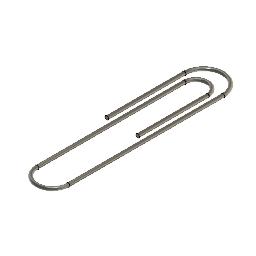
Semana2_Desafio5 v1 (Autodesk Fusion 360 design; units mm, degrees)
Autodesk Fusion 360 part; units mm, degrees
sketch "Sketch6" plane through (0, 0, 0) normal (0, 0, 1) x (1, 0, 0)
  line L0 (0, 0) -> (0, 50)
  arc A0 (25, 50) -> (0, 50) centre (12.5, 50) ccw
  line L1 (25, 50) -> (25, -50)
  arc A1 (5, -50) -> (25, -50) centre (15, -50) ccw
  line L2 (5, -50) -> (5, 45)
  arc A2 (20, 45) -> (5, 45) centre (12.5, 45) ccw
  line L3 (20, 45) -> (20, 0)
  constraint coincident L0.start origin
  constraint vertical L0
  constraint tangent L0 A0
  constraint tangent A0 L1
  constraint parallel L0 L1
  constraint tangent L1 A1
  constraint tangent A1 L2
  constraint parallel L1 L2
  constraint tangent L2 A2
  constraint tangent A2 L3
  constraint parallel L2 L3
sketch "Sketch8" plane through (0, 0, 0) normal (0, 1, 0) x (1, 0, 0)
  circle A0 centre (0, 0) radius 1.25
  dimension "d4" = 2.5
  constraint coincident A0.centre origin
  measures "d4" diameter of A0
sweep "Sweep1" add profiles "Sketch8" path "Sketch6" along L0 A0 L1 A1 L2 A2 L3 section 1
